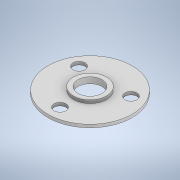
# Autodesk Inventor part: CircSpacer
Saved by Autodesk Inventor 2022.2 (Build 262287030, 287C)
## iProperties
Created: 2023-02-08
Part Number: CircSpacer
Material: Generic
Document SubType Name: Modeling
Designer: jak27277
Density: 1 g/cm^3
Appearance: Default
Author: jak27277
Autodesk Inventor part; units mm, degrees
ref_plane "YZ Plane" through (0, 0, 0) normal (1, 0, 0) x (0, 1, 0)
ref_plane "XZ Plane" through (0, 0, 0) normal (0, 1, 0) x (-1, 0, 0)
ref_plane "XY Plane" through (0, 0, 0) normal (0, 0, 1) x (1, 0, 0)
sketch "Sketch1" plane through (0, 0, 0) normal (0, 1, 0) x (-1, 0, 0)
  circle A0 centre (0, 0) radius 88.9
  circle A1 centre (0, 0) radius 25.4
  circle A2 centre (0, 0) radius 34.925
  line L0 (0, 0) -> (0, 63.5) construction
  circle A3 centre (0, 63.5) radius 12.7
  line L1 (0, 0) -> (-54.9926, -31.75) construction
  circle A4 centre (-54.9926, -31.75) radius 12.7
  line L2 (0, 0) -> (54.9926, -31.75) construction
  circle A5 centre (54.9926, -31.75) radius 12.7
  dimension "d0" = 177.8
  dimension "d1" = 25.4
  dimension "d2" = 63.5
  dimension "d3" = 69.85
  dimension "d4" = 50.8
  dimension "d7" = 360
  constraints: 6 centre point, 6 coincident, 6 end point, 1 vertical, 16 other
  measures "d0" diameter of A0
  measures "d1" diameter of A3
  measures "d2" distance of L0.start L0.end
  measures "d3" diameter of A2
  measures "d4" diameter of A1
extrude "Extrusion1" add sketch "Sketch1" along normal blind 6.35 contours A0 | A2
sketch "Sketch3" plane through (0, 6.35, 0) normal (0, 1, 0) x (1, 0, 0)
  circle A0 centre (0, 0) radius 88.9 projected
  circle A1 centre (-54.9926, 31.75) radius 12.7 projected
  circle A2 centre (54.9926, 31.75) radius 12.7 projected
  circle A3 centre (0, -63.5) radius 12.7 projected
  circle A4 centre (0, 0) radius 34.925
  circle A5 centre (0, 0) radius 25.4 projected
  circle A6 centre (0, 0) radius 25.4
  dimension "d11" = 69.85
  dimension "d14" = 50.8
  constraints: 2 centre point, 2 coincident
  measures "d11" diameter of A4
  measures "d14" diameter of A5
extrude "Extrusion2" add sketch "Sketch3" along normal blind 6.35 contours A4
body "Solid1"
